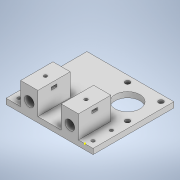
# Autodesk Inventor part: HalterungMotorNeu
Saved by Autodesk Inventor 2021 (Build 250183000, 183)
## iProperties
Created: 2021-02-28
Part Number: HalterungMotorNeu
Material: Generisch
Document SubType Name: Modeling
Designer: Elena
Density: 1 g/cm^3
Appearance: Vorgabe
Author: Elena
Autodesk Inventor part; units mm, degrees
ref_plane "YZ Plane" through (0, 0, 0) normal (1, 0, 0) x (0, 1, 0)
ref_plane "XZ Plane" through (0, 0, 0) normal (0, 1, 0) x (-1, 0, 0)
ref_plane "XY Plane" through (0, 0, 0) normal (0, 0, 1) x (1, 0, 0)
sketch "Skizze1" plane through (0, 0, 0) normal (0, 1, 0) x (-1, 0, 0)
  line L0 (0, 0) -> (65.65, 0)
  line L1 (65.65, 0) -> (65.65, -80)
  line L2 (65.65, -80) -> (0, -80)
  line L3 (0, -80) -> (0, 0)
  dimension "d0" = 65.65
  dimension "d1" = 80
  constraints: 8 end point, 2 parallel, 1 horizontal, 1 perpendicular
  measures "d0" distance of L1.end L2.end
  measures "d1" distance of L0.end L1.end
extrude "Extrusion1" add sketch "Skizze1" along normal blind 5
sketch "Skizze2" plane through (0, 5, 0) normal (0, 1, 0) x (1, 0, 0)
  line L0 (-65.65, 80) -> (-65.65, 0) projected
  line L1 (-65.65, 0) -> (0, 0) projected
  line L2 (-65.65, 0) -> (-59.65, 0) construction
  line L3 (-59.65, 0) -> (-59.65, 30)
  line L4 (-59.65, 30) -> (-43.65, 30)
  line L5 (-43.65, 30) -> (-43.65, 0)
  line L6 (-43.65, 0) -> (-59.65, 0)
  line L7 (-22, 0) -> (-22, 30)
  line L8 (-22, 30) -> (-6, 30)
  line L9 (-6, 30) -> (-6, 0)
  line L10 (-6, 0) -> (-22, 0)
  dimension "d4" = 6
  dimension "d6" = 30
  dimension "d7" = 16
  dimension "d8" = 90
  dimension "d9" = 16
  dimension "d10" = 21.65
  dimension "d11" = 30
  dimension "d12" = 16
  dimension "d13" = 90
  dimension "d14" = 30
  dimension "d15" = 90
  constraints: 18 end point, 5 perpendicular, 2 point on line, 1 collinear, 1 horizontal
  measures "d4" distance of L0.end L3.start
  measures "d6" distance of L3.start L3.end
  measures "d7" distance of L3.end L4.end
  measures "d8" angle of L3 L4
  measures "d9" distance of L5.end L3.start
  measures "d10" distance of L5.end L7.start
  measures "d11" distance of L7.start L7.end
  measures "d12" distance of L7.end L8.end
  measures "d13" angle of L7 L8
  measures "d14" distance of L8.end L9.end
  measures "d15" angle of L8 L9
extrude "Extrusion2" add sketch "Skizze2" along normal blind 21 contours L3 L4 L5 L1
sketch "Skizze3" plane through (0, 5, 0) normal (0, 1, 0) x (1, 0, 0)
  line L0 (-43.65, 0) -> (0, 0) projected
  line L1 (-43.65, 0) -> (-22, 0)
  line L2 (-22, 0) -> (-22, 30)
  line L3 (-22, 30) -> (-6, 30)
  line L4 (-6, 30) -> (-6, 0)
  line L5 (-6, 0) -> (-22, 0)
  dimension "d18" = 21.65
  dimension "d19" = 30
  dimension "d21" = 16
  dimension "d22" = 16
  constraints: 10 end point, 2 perpendicular, 2 point on line, 1 collinear, 1 horizontal
  measures "d18" distance of L0.start L1.end
  measures "d19" distance of L1.end L2.end
  measures "d21" distance of L2.end L3.end
  measures "d22" distance of L4.end L1.end
extrude "Extrusion3" add sketch "Skizze3" along normal blind 21
sketch "Skizze4" plane through (0, 5, 0) normal (0, 1, 0) x (1, 0, 0)
  line L0 (-65.65, 0) -> (0, 0) projected
  line L1 (-5.9719, 0) -> (14.5281, 0)
  line L2 (14.5281, 0) -> (14.5281, 80)
  line L3 (0, 0) -> (0, 80) projected
  line L4 (14.5281, 80) -> (0, 80)
  line L5 (0, 80) -> (0, 0)
  dimension "d25" = 20.5
  dimension "d26" = 80
  dimension "d27" = 90
  constraints: 8 end point, 2 perpendicular, 1 collinear, 1 point on line
  measures "d25" distance of L1.start L1.end
  measures "d26" distance of L1.end L2.end
  measures "d27" angle of L2 L1
extrude "Extrusion4" add sketch "Skizze4" against normal blind 5
sketch "Skizze5" plane through (0, 5, 0) normal (0, 1, 0) x (1, 0, 0)
  line L0 (-22, 30) -> (-6, 30) projected
  line L1 (-22, 30) -> (-14, 30)
  line L2 (-14, 30) -> (-14, 38)
  line L3 (-14, 38) -> (-29.5, 38)
  circle A0 centre (-29.5, 38) radius 1
  point P0 (0, 0)
  dimension "d30" = 8
  dimension "d31" = 8
  dimension "d32" = 15.5
  dimension "d33" = 2
  constraints: 6 end point, 2 perpendicular, 1 centre point, 1 coincident, 1 midpoint
  measures "d30" distance of L0.start L1.end
  measures "d31" distance of L1.end L2.end
  measures "d32" distance of L2.end L3.end
  measures "d33" diameter of A0
extrude "Extrusion5" cut sketch "Skizze5" against normal blind 5
sketch "Skizze6" plane through (0, 5, 0) normal (0, 1, 0) x (1, 0, 0)
  circle A0 centre (-29.5, 38) radius 1 projected
  line L0 (-29.5, 38) -> (1.5, 38)
  line L1 (-29.5, 38) -> (1.5, 38) construction
  circle A1 centre (1.5, 38) radius 1
  point P0 (0, 0)
  dimension "d36" = 31
  dimension "d37" = 0
  dimension "d38" = 2
  constraints: 4 end point, 2 horizontal, 1 centre point, 1 coincident, 1 collinear
  measures "d36" distance of L0.start L0.end
  measures "d37" distance between parallel lines of L0 L1
  measures "d38" diameter of A1
extrude "Extrusion6" cut sketch "Skizze6" against normal blind 5 contours A1
sketch "Skizze7" plane through (0, 5, 0) normal (0, 1, 0) x (1, 0, 0)
  circle A0 centre (1.5, 38) radius 1 projected
  line L0 (1.5, 38) -> (1.5, 69)
  circle A1 centre (1.5, 69) radius 1
  point P0 (0, 0)
  dimension "d41" = 31
  dimension "d42" = 2
  constraints: 2 end point, 1 centre point, 1 coincident, 1 vertical
  measures "d41" distance of L0.start L0.end
  measures "d42" diameter of A1
extrude "Extrusion7" cut sketch "Skizze7" against normal blind 5 contours A1
sketch "Skizze8" plane through (0, 5, 0) normal (0, 1, 0) x (1, 0, 0)
  circle A0 centre (-29.5, 38) radius 1 projected
  line L0 (-29.5, 38) -> (-29.5, 69)
  circle A1 centre (-29.5, 69) radius 1
  point P0 (0, 0)
  dimension "d45" = 31
  dimension "d46" = 2
  constraints: 2 end point, 1 centre point, 1 coincident, 1 vertical
  measures "d45" distance of L0.start L0.end
  measures "d46" diameter of A1
extrude "Extrusion8" cut sketch "Skizze8" against normal blind 5 contours A1
sketch "Skizze9" plane through (0, 5, 0) normal (0, 1, 0) x (1, 0, 0)
  circle A0 centre (1.5, 38) radius 1 projected
  line L0 (1.5, 38) -> (7.5, 38)
  line L1 (14.5281, 80) -> (-65.65, 80) projected
  line L2 (-65.65, 0) -> (14.5281, 0) projected
  line L3 (14.5281, 0) -> (14.5281, 80) projected
  line L4 (7.5, 38) -> (14.5281, 38)
  line L5 (14.5281, 38) -> (14.5281, 80)
  line L6 (14.5281, 80) -> (7.5, 80)
  line L7 (7.5, 80) -> (7.5, 38)
  point P0 (0, 0)
  dimension "d49" = 6
  constraints: 10 end point, 2 horizontal, 2 parallel, 1 perpendicular
  measures "d49" distance of L0.start L0.end
extrude "Extrusion9" cut sketch "Skizze9" against normal blind 5 contours L7 L1 L3 L4
sketch "Skizze10" plane through (0, 5, 0) normal (0, 1, 0) x (1, 0, 0)
  line L0 (7.5, 38) -> (7.5, 80) projected
  line L1 (14.5281, 0) -> (14.5281, 38) projected
  line L2 (7.5, 38) -> (14.5281, 38)
  line L3 (14.5281, 38) -> (14.5281, 0)
  line L4 (14.5281, 0) -> (7.5, 0)
  line L5 (7.5, 0) -> (7.5, 38)
  point P0 (0, 0)
  constraints: 8 end point, 2 parallel, 1 horizontal, 1 perpendicular
extrude "Extrusion10" cut sketch "Skizze10" against normal blind 5
sketch "Skizze11" plane through (0, 5, 0) normal (0, 1, 0) x (1, 0, 0)
  circle A0 centre (1.5, 69) radius 1 projected
  line L0 (1.5, 69) -> (1.5, 75)
  line L1 (1.5, 75) -> (7.5, 75)
  line L2 (7.5, 0) -> (7.5, 80) projected
  line L3 (7.5, 80) -> (1.5, 80)
  line L4 (7.5, 80) -> (-65.65, 80) projected
  line L5 (1.5, 75) -> (1.5, 80)
  point P0 (0, 0)
  dimension "d54" = 6
  constraints: 8 end point, 3 point on line, 2 perpendicular, 1 vertical
  measures "d54" distance of L0.start L0.end
extrude "Extrusion11" cut sketch "Skizze11" against normal blind 5 contours L5 L3 L2 L1
sketch "Skizze12" plane through (0, 5, 0) normal (0, 1, 0) x (1, 0, 0)
  line L0 (1.5, 80) -> (-65.65, 80) projected
  line L1 (1.5, 75) -> (-65.65, 75)
  line L2 (-65.65, 75) -> (-65.65, 80)
  line L3 (-65.65, 80) -> (1.5, 80)
  line L4 (1.5, 80) -> (1.5, 75)
  point P0 (0, 0)
  constraints: 8 end point, 2 parallel, 1 horizontal, 1 perpendicular
extrude "Extrusion12" cut sketch "Skizze12" against normal blind 5
sketch "Skizze13" plane through (0, 5, 0) normal (0, 1, 0) x (1, 0, 0)
  circle A0 centre (1.5, 38) radius 1 projected
  line L0 (1.5, 38) -> (1.5, 23)
  circle A1 centre (1.5, 23) radius 1
  point P0 (0, 0)
  dimension "d59" = 15
  dimension "d60" = 2
  constraints: 2 end point, 1 centre point, 1 coincident, 1 vertical
  measures "d59" distance of L0.start L0.end
  measures "d60" diameter of A1
extrude "Extrusion13" cut sketch "Skizze13" against normal blind 5 contours A1
sketch "Skizze14" plane through (0, 5, 0) normal (0, 1, 0) x (1, 0, 0)
  circle A0 centre (1.5, 23) radius 1 projected
  line L0 (-65.65, 0) -> (7.5, 0) projected
  line L1 (-6, 30) -> (-6, 0) projected
  line L2 (1.5, 0) -> (-6, 0)
  line L3 (1.5, 0) -> (1.5, 6)
  circle A1 centre (1.5, 6) radius 1
  point P0 (0, 0)
  dimension "d63" = 6
  dimension "d64" = 2
  constraints: 4 end point, 1 centre point, 1 coincident, 1 horizontal, 1 point on line, 1 vertical
  measures "d63" distance of L2.start L3.end
  measures "d64" diameter of A1
extrude "Extrusion14" cut sketch "Skizze14" against normal blind 5 contours A1
sketch "Skizze15" plane through (0, 5, 0) normal (0, 1, 0) x (1, 0, 0)
  line L0 (-65.65, 0) -> (7.5, 0) projected
  line L1 (-65.65, 0) -> (-62.65, 0)
  line L2 (-62.65, 0) -> (-62.65, 6)
  circle A0 centre (-62.65, 6) radius 1
  point P0 (0, 0)
  dimension "d67" = 3
  dimension "d68" = 6
  dimension "d69" = 2
  constraints: 4 end point, 1 centre point, 1 coincident, 1 perpendicular, 1 point on line
  measures "d67" distance of L0.start L1.end
  measures "d68" distance of L1.end L2.end
  measures "d69" diameter of A0
extrude "Extrusion15" cut sketch "Skizze15" against normal blind 5
sketch "Skizze16" plane through (0, 5, 0) normal (0, 1, 0) x (1, 0, 0)
  circle A0 centre (-62.65, 6) radius 1 projected
  line L0 (-62.65, 6) -> (-62.65, 23)
  circle A1 centre (-62.65, 23) radius 1
  point P0 (0, 0)
  dimension "d72" = 17
  dimension "d73" = 2
  constraints: 2 end point, 1 centre point, 1 coincident, 1 vertical
  measures "d72" distance of L0.start L0.end
  measures "d73" diameter of A1
extrude "Extrusion16" cut sketch "Skizze16" against normal blind 5 contours A1
sketch "Skizze17" plane through (-65.65, 0, 0) normal (0, 0, 1) x (1, 0, 0)
  line L0 (6, 26) -> (22, 26) projected
  line L1 (6, 26) -> (14, 26)
  line L2 (14, 26) -> (14, 13)
  circle A0 centre (14, 13) radius 4.5
  point P0 (65.65, 0)
  dimension "d76" = 8
  dimension "d77" = 13
  dimension "d78" = 9
  constraints: 4 end point, 1 centre point, 1 coincident, 1 midpoint, 1 perpendicular
  measures "d76" distance of L0.start L1.end
  measures "d77" distance of L1.end L2.end
  measures "d78" diameter of A0
extrude "Extrusion17" cut sketch "Skizze17" against normal blind 30
sketch "Skizze18" plane through (-65.65, 0, 0) normal (0, 0, 1) x (1, 0, 0)
  line L0 (43.65, 5) -> (43.65, 26) projected
  line L1 (43.65, 26) -> (51.65, 26)
  line L2 (51.65, 26) -> (51.65, 13)
  circle A0 centre (51.65, 13) radius 4.5
  point P0 (65.65, 0)
  dimension "d81" = 8
  dimension "d82" = 13
  dimension "d83" = 9
  constraints: 4 end point, 1 centre point, 1 coincident, 1 horizontal, 1 perpendicular
  measures "d81" distance of L0.end L1.end
  measures "d82" distance of L1.end L2.end
  measures "d83" diameter of A0
extrude "Extrusion18" cut sketch "Skizze18" against normal blind 30
sketch "Skizze19" plane through (-59.65, 5, -30) normal (-1, 0, 0) x (0, 0, 1)
  line L0 (0, 0) -> (0, 21) projected
  line L1 (0, 21) -> (15, 21)
  line L2 (0, 21) -> (30, 21) projected
  line L3 (15, 21) -> (15, 17)
  line L4 (15, 17) -> (17.75, 17)
  line L5 (17.75, 17) -> (12.25, 17)
  line L6 (12.25, 17) -> (12.25, 15.75)
  line L7 (12.25, 15.75) -> (17.75, 15.75)
  line L8 (17.75, 15.75) -> (17.75, 17)
  point P0 (30, -5)
  dimension "d86" = 15
  dimension "d87" = 4
  dimension "d88" = 2.75
  dimension "d89" = 5.5
  dimension "d90" = 1.25
  constraints: 14 end point, 3 perpendicular, 2 parallel, 1 horizontal, 1 midpoint
  measures "d86" distance of L0.end L1.end
  measures "d87" distance of L1.end L3.end
  measures "d88" distance of L3.end L4.end
  measures "d89" distance of L7.end L6.end
  measures "d90" distance of L6.end L5.end
extrude "Extrusion19" cut sketch "Skizze19" against normal blind 16
sketch "Skizze20" plane through (0, 5, 0) normal (0, 1, 0) x (1, 0, 0)
  circle A0 centre (1.5, 23) radius 1 projected
  circle A1 centre (1.5, 23) radius 1.5
  point P0 (0, 0)
  dimension "d93" = 3
  constraints: 1 centre point, 1 coincident
  measures "d93" diameter of A1
extrude "Extrusion20" cut sketch "Skizze20" against normal blind 5 contours A0 | A1
sketch "Skizze21" plane through (0, 5, 0) normal (0, 1, 0) x (1, 0, 0)
  circle A0 centre (1.5, 6) radius 1 projected
  circle A1 centre (1.5, 6) radius 1.5
  point P0 (0, 0)
  dimension "d96" = 3
  constraints: 1 centre point, 1 coincident
  measures "d96" diameter of A1
extrude "Extrusion21" cut sketch "Skizze21" against normal blind 5 contours A0 | A1
sketch "Skizze22" plane through (0, 5, 0) normal (0, 1, 0) x (1, 0, 0)
  circle A0 centre (-62.65, 23) radius 1 projected
  circle A1 centre (-62.65, 23) radius 1.5
  point P0 (0, 0)
  dimension "d99" = 3
  constraints: 1 centre point, 1 coincident
  measures "d99" diameter of A1
extrude "Extrusion22" cut sketch "Skizze22" against normal blind 5 contours A0 | A1
sketch "Skizze23" plane through (0, 5, 0) normal (0, 1, 0) x (1, 0, 0)
  circle A0 centre (-62.65, 6) radius 1 projected
  circle A1 centre (-62.65, 6) radius 1.5
  point P0 (0, 0)
  dimension "d102" = 3
  constraints: 1 centre point, 1 coincident
  measures "d102" diameter of A1
extrude "Extrusion23" cut sketch "Skizze23" against normal blind 5 contours A0 | A1
sketch "Skizze24" plane through (0, 5, 0) normal (0, 1, 0) x (1, 0, 0)
  circle A0 centre (1.5, 69) radius 1 projected
  circle A1 centre (1.5, 69) radius 2.25
  point P0 (0, 0)
  dimension "d105" = 4.5
  constraints: 1 centre point, 1 coincident
  measures "d105" diameter of A1
extrude "Extrusion24" cut sketch "Skizze24" against normal blind 5 contours A0 | A1
sketch "Skizze25" plane through (0, 5, 0) normal (0, 1, 0) x (1, 0, 0)
  circle A0 centre (-29.5, 69) radius 1 projected
  circle A1 centre (-29.5, 69) radius 2.25
  point P0 (0, 0)
  dimension "d108" = 4.5
  constraints: 1 centre point, 1 coincident
  measures "d108" diameter of A1
extrude "Extrusion25" cut sketch "Skizze25" against normal blind 5 contours A0 | A1
sketch "Skizze26" plane through (0, 5, 0) normal (0, 1, 0) x (1, 0, 0)
  circle A0 centre (1.5, 38) radius 1 projected
  circle A1 centre (1.5, 38) radius 2.25
  point P0 (0, 0)
  dimension "d112" = 4.5
  constraints: 1 centre point, 1 coincident
  measures "d112" diameter of A1
extrude "Extrusion26" cut sketch "Skizze26" against normal blind 5 contours A0 | A1
sketch "Skizze27" plane through (0, 5, 0) normal (0, 1, 0) x (1, 0, 0)
  circle A0 centre (-29.5, 38) radius 1 projected
  circle A1 centre (-29.5, 38) radius 2.25
  point P0 (0, 0)
  dimension "d115" = 4.5
  constraints: 1 centre point, 1 coincident
  measures "d115" diameter of A1
extrude "Extrusion27" cut sketch "Skizze27" against normal blind 5 contours A0 | A1
sketch "Skizze28" plane through (0, 26, 0) normal (0, 1, 0) x (1, 0, 0)
  line L0 (-43.65, 30) -> (-43.65, 0) projected
  line L1 (-59.65, 0) -> (-59.65, 30) projected
  line L2 (-43.65, 0) -> (-59.65, 30)
  line L3 (-59.65, 30) -> (-43.65, 30) projected
  line L4 (-43.65, 30) -> (-59.65, 0)
  circle A0 centre (-51.65, 15) radius 1.5
  point P0 (0, 0)
  dimension "d118" = 3
  constraints: 4 end point, 1 centre point, 1 midpoint
  measures "d118" diameter of A0
extrude "Extrusion28" cut sketch "Skizze28" against normal blind 13 contours A0 L2 L4 | L4 L2 A0 | A0 L4 L2 | L2 L4 A0
sketch "Skizze29" plane through (-6, 5, 0) normal (1, 0, 0) x (0, 0, -1)
  line L0 (0, 21) -> (15, 21)
  line L1 (0, 21) -> (30, 21) projected
  line L2 (15, 21) -> (11, 21)
  line L3 (15, 21) -> (15, 17)
  line L4 (15, 21) -> (19, 21) construction
  line L5 (15, 17) -> (17.27, 17)
  line L6 (12.25, 17) -> (17.75, 17) projected
  line L7 (17.27, 17) -> (11.77, 17)
  line L8 (11.77, 17) -> (11.77, 15.75)
  line L9 (11.77, 15.75) -> (17.27, 15.75)
  line L10 (17.27, 15.75) -> (17.27, 17)
  point P0 (0, -5)
  dimension "d123" = 15
  dimension "d124" = 4
  dimension "d125" = 4
  dimension "d126" = 90
  dimension "d127" = 2.27
  dimension "d128" = 5.5
  dimension "d129" = 1.25
  constraints: 18 end point, 2 horizontal, 2 parallel, 2 perpendicular, 2 point on line, 1 midpoint, 1 vertical
  measures "d123" distance of L0.start L0.end
  measures "d124" distance of L0.end L2.end
  measures "d125" distance of L0.end L3.end
  measures "d126" angle of L3 L4
  measures "d127" distance of L3.end L5.end
  measures "d128" distance of L9.end L8.end
  measures "d129" distance of L8.end L7.end
extrude "Extrusion29" cut sketch "Skizze29" against normal blind 16
sketch "Skizze30" plane through (0, 26, 0) normal (0, 1, 0) x (1, 0, 0)
  line L0 (-22, 30) -> (-22, 0) projected
  line L1 (-6, 0) -> (-6, 30) projected
  line L2 (-22, 0) -> (-6, 30)
  line L3 (-22, 30) -> (-6, 0)
  circle A0 centre (-14, 15) radius 1.5
  point P0 (0, 0)
  dimension "d132" = 3
  constraints: 4 end point, 1 centre point, 1 midpoint
  measures "d132" diameter of A0
extrude "Extrusion30" cut sketch "Skizze30" against normal blind 13 contours A0 L2 L3 | L3 L2 A0 | L2 L3 A0 | L2 A0 L3
sketch "Skizze31" plane through (0, 5, 0) normal (0, 1, 0) x (1, 0, 0)
  circle A0 centre (-29.5, 38) radius 2.25 projected
  circle A1 centre (1.5, 69) radius 2.25 projected
  line L0 (-29.5, 38) -> (1.5, 69)
  circle A2 centre (-29.5, 69) radius 2.25 projected
  circle A3 centre (1.5, 38) radius 2.25 projected
  line L1 (-29.5, 69) -> (1.5, 38)
  circle A4 centre (-14, 53.5) radius 11.5
  point P0 (0, 0)
  dimension "d137" = 23
  constraints: 4 end point, 1 centre point, 1 midpoint
  measures "d137" diameter of A4
extrude "Extrusion31" cut sketch "Skizze31" against normal blind 5 contours A4 L1 L0 | L0 L1 A4 | L1 A4 L0 | L0 A4 L1
sketch "Skizze32" plane through (0, 5, 0) normal (0, 1, 0) x (1, 0, 0)
  point P0 (0, 0)
sketch "Skizze33" plane through (0, 5, 0) normal (0, 1, 0) x (1, 0, 0)
  circle A0 centre (-62.65, 6) radius 1.5 projected
  circle A1 centre (-62.65, 6) radius 1.5
  point P0 (0, 0)
  dimension "d140" = 3
  constraints: 1 centre point, 1 coincident
  measures "d140" diameter of A1
extrude "Extrusion32" add sketch "Skizze33" against normal blind 5
sketch "Skizze34" plane through (0, 5, 0) normal (0, 1, 0) x (1, 0, 0)
  circle A0 centre (-62.65, 23) radius 1.5 projected
  circle A1 centre (-62.65, 23) radius 1.5
  point P0 (0, 0)
  dimension "d143" = 3
  constraints: 1 centre point, 1 coincident
  measures "d143" diameter of A1
extrude "Extrusion33" add sketch "Skizze34" against normal blind 5
sketch "Skizze35" plane through (0, 5, 0) normal (0, 1, 0) x (1, 0, 0)
  line L0 (-59.65, 0) -> (-59.65, 30) projected
  line L1 (-59.65, 0) -> (-73.15, 0)
  line L2 (-65.65, 0) -> (-59.65, 0) projected
  line L3 (-65.65, 0) -> (7.5, 0) projected
  line L4 (-65.65, 0) -> (-73.15, 0)
  line L5 (-73.15, 0) -> (-73.15, 75)
  line L6 (-73.15, 75) -> (-65.65, 75)
  line L7 (-65.65, 75) -> (-65.65, 0)
  point P0 (0, 0)
  dimension "d146" = 13.5
  dimension "d147" = 75
  constraints: 10 end point, 2 parallel, 1 collinear, 1 horizontal, 1 perpendicular
  measures "d146" distance of L0.start L1.end
  measures "d147" distance of L4.end L5.end
extrude "Extrusion34" add sketch "Skizze35" against normal blind 5
sketch "Skizze36" plane through (0, 5, 0) normal (0, 1, 0) x (1, 0, 0)
  line L0 (-73.15, 0) -> (-73.15, 75) projected
  line L1 (-73.15, 0) -> (-67.15, 0)
  line L2 (-67.15, 0) -> (-67.15, 6)
  line L3 (-67.15, 6) -> (-73.15, 6)
  line L4 (-73.15, 6) -> (-73.15, 0)
  circle A0 centre (-67.15, 6) radius 1.5
  point P0 (0, 0)
  dimension "d150" = 6
  dimension "d151" = 6
  dimension "d152" = 3
  constraints: 8 end point, 2 parallel, 1 centre point, 1 coincident, 1 horizontal, 1 perpendicular
  measures "d150" distance of L3.end L2.end
  measures "d151" distance of L2.end L1.end
  measures "d152" diameter of A0
extrude "Extrusion35" cut sketch "Skizze36" against normal blind 5 contours A0 L2 L3 | L3 L2 A0
sketch "Skizze37" plane through (0, 5, 0) normal (0, 1, 0) x (1, 0, 0)
  circle A0 centre (-67.15, 6) radius 1.5 projected
  line L0 (-67.15, 6) -> (-67.15, 23)
  circle A1 centre (-67.15, 23) radius 1.5
  point P0 (0, 0)
  dimension "d155" = 17
  dimension "d156" = 3
  constraints: 2 end point, 1 centre point, 1 coincident, 1 vertical
  measures "d155" distance of L0.start L0.end
  measures "d156" diameter of A1
extrude "Extrusion36" cut sketch "Skizze37" against normal blind 5 contours A1
sketch "Skizze38" plane through (-6, 5, 0) normal (1, 0, 0) x (0, 0, -1)
  line L0 (17.27, 17) -> (11.77, 17) projected
  line L1 (11.77, 17) -> (11.77, 17.625)
  line L2 (11.77, 17.625) -> (17.27, 17.625)
  line L3 (17.27, 17.625) -> (17.27, 17)
  line L4 (12.25, 17) -> (17.75, 17) projected
  point P0 (0, -5)
  dimension "d159" = 0.625
  dimension "d160" = 5.5
  dimension "d161" = 90
  constraints: 6 end point, 2 perpendicular, 1 point on line, 1 vertical
  measures "d159" distance of L0.end L1.end
  measures "d160" distance of L1.end L2.end
  measures "d161" angle of L1 L2
extrude "Extrusion37" cut sketch "Skizze38" against normal blind 16
sketch "Skizze39" plane through (-6, 5, 0) normal (1, 0, 0) x (0, 0, -1)
  line L0 (17.27, 15.75) -> (11.77, 15.75) projected
  line L1 (11.77, 15.75) -> (17.27, 15.75)
  line L2 (17.27, 15.75) -> (17.27, 15.125)
  line L3 (17.27, 15.125) -> (11.77, 15.125)
  line L4 (11.77, 15.125) -> (11.77, 15.75)
  point P0 (0, -5)
  dimension "d164" = 5.5
  dimension "d165" = 0.625
  constraints: 8 end point, 2 parallel, 1 horizontal, 1 perpendicular
  measures "d164" distance of L2.end L3.end
  measures "d165" distance of L1.end L2.end
extrude "Extrusion38" cut sketch "Skizze39" against normal blind 16
sketch "Skizze40" plane through (-59.65, 5, -30) normal (-1, 0, 0) x (0, 0, 1)
  line L0 (12.73, 17.625) -> (18.23, 17.625) projected
  line L1 (12.25, 17) -> (17.75, 17)
  line L2 (17.75, 17) -> (17.75, 17.625)
  line L3 (17.75, 17.625) -> (12.25, 17.625)
  line L4 (12.25, 17.625) -> (12.25, 17)
  point P0 (30, -5)
  dimension "d168" = 5.5
  constraints: 8 end point, 2 parallel, 1 horizontal, 1 perpendicular, 1 point on line
  measures "d168" distance of L3.end L2.end
extrude "Extrusion39" cut sketch "Skizze40" against normal blind 16
sketch "Skizze41" plane through (-59.65, 5, -30) normal (-1, 0, 0) x (0, 0, 1)
  line L0 (12.25, 15.75) -> (17.75, 15.75) projected
  line L1 (12.25, 15.75) -> (17.75, 15.75)
  line L2 (17.75, 15.75) -> (17.75, 15.125)
  line L3 (17.75, 15.125) -> (12.25, 15.125)
  line L4 (12.25, 15.125) -> (12.25, 15.75)
  point P0 (30, -5)
  dimension "d171" = 5.5
  dimension "d172" = 0.625
  constraints: 8 end point, 2 parallel, 1 horizontal, 1 perpendicular
  measures "d171" distance of L2.end L3.end
  measures "d172" distance of L1.end L2.end
extrude "Extrusion40" cut sketch "Skizze41" against normal blind 16
sketch "Skizze42" plane through (-6, 5, 0) normal (1, 0, 0) x (0, 0, -1)
  line L0 (11.77, 17.625) -> (11.77, 15.125) projected
  line L1 (17.75, 15.125) -> (12.25, 15.125) projected
  line L2 (11.77, 17.625) -> (17.27, 17.625)
  line L3 (17.27, 17.625) -> (17.27, 15.125)
  line L4 (17.27, 15.125) -> (11.77, 15.125)
  line L5 (11.77, 15.125) -> (11.77, 17.625)
  point P0 (0, -5)
  dimension "d175" = 5.5
  constraints: 8 end point, 2 parallel, 1 horizontal, 1 perpendicular, 1 point on line
  measures "d175" distance of L3.end L4.end
extrude "Extrusion41" add sketch "Skizze42" against normal blind 16
sketch "Skizze43" plane through (0, 26, 0) normal (0, 1, 0) x (1, 0, 0)
  circle A0 centre (-14, 15) radius 1.5 projected
  line L0 (-14, 15) -> (-6, 15)
  line L1 (-6, 0) -> (-6, 30) projected
  point P0 (0, 0)
  constraints: 2 end point, 1 midpoint
sketch "Skizze44" plane through (-6, 5, 0) normal (1, 0, 0) x (0, 0, -1)
  line L0 (0, 21) -> (30, 21) projected
  line L1 (15, 21) -> (15, 17.5)
  line L2 (15, 17.5) -> (17.55, 17.5)
  line L3 (17.55, 17.5) -> (17.55, 15)
  line L4 (17.55, 15) -> (12.45, 15)
  line L5 (12.45, 15) -> (12.45, 17.5)
  line L6 (12.45, 17.5) -> (15, 17.5)
  point P0 (0, -5)
  dimension "d178" = 3.5
  dimension "d179" = 2.55
  dimension "d180" = 2.5
  dimension "d181" = 90
  dimension "d182" = 5.1
  dimension "d183" = 2.5
  constraints: 12 end point, 3 perpendicular, 1 midpoint, 1 point on line, 1 vertical
  measures "d178" distance of L1.start L1.end
  measures "d179" distance of L1.end L2.end
  measures "d180" distance of L2.end L3.end
  measures "d181" angle of L2 L3
  measures "d182" distance of L3.end L4.end
  measures "d183" distance of L4.end L5.end
extrude "Extrusion42" cut sketch "Skizze44" against normal blind 16
sketch "Skizze45" plane through (0, 26, 0) normal (0, 1, 0) x (1, 0, 0)
  circle A0 centre (-14, 15) radius 1.5 projected
  circle A1 centre (-14, 15) radius 1.5
  point P0 (0, 0)
  dimension "d186" = 3
  constraints: 1 centre point, 1 coincident
  measures "d186" diameter of A1
extrude "Extrusion43" add sketch "Skizze45" against normal blind 3.6
extrude "Extrusion44" cut sketch "Skizze43" against normal blind 3.6
sketch "Skizze46" plane through (-59.65, 5, -30) normal (-1, 0, 0) x (0, 0, 1)
  line L0 (12.25, 17.625) -> (12.25, 15.125) projected
  line L1 (12.25, 15.125) -> (17.75, 15.125) projected
  line L2 (12.25, 17.625) -> (17.75, 17.625)
  line L3 (17.75, 17.625) -> (17.75, 15.125)
  line L4 (17.75, 15.125) -> (12.25, 15.125)
  line L5 (12.25, 15.125) -> (12.25, 17.625)
  point P0 (30, -5)
  constraints: 8 end point, 2 parallel, 1 horizontal, 1 perpendicular
extrude "Extrusion45" add sketch "Skizze46" against normal blind 16
sketch "Skizze47" plane through (0, 26, 0) normal (0, 1, 0) x (1, 0, 0)
  circle A0 centre (-51.65, 15) radius 1.5 projected
  line L0 (-51.65, 15) -> (-59.65, 15)
  line L1 (-59.65, 30) -> (-59.65, 0) projected
  point P0 (0, 0)
  constraints: 2 end point, 1 midpoint
sketch "Skizze48" plane through (-59.65, 5, -30) normal (-1, 0, 0) x (0, 0, 1)
  line L0 (0, 21) -> (30, 21) projected
  line L1 (15, 21) -> (15, 17.5)
  line L2 (15, 21) -> (18.5, 21) construction
  line L3 (15, 17.5) -> (17.55, 17.5)
  line L4 (17.55, 17.5) -> (17.55, 15)
  line L5 (17.55, 15) -> (12.45, 15)
  line L6 (12.45, 15) -> (12.45, 17.5)
  line L7 (12.45, 17.5) -> (15, 17.5)
  point P0 (30, -5)
  dimension "d193" = 3.5
  dimension "d194" = 90
  dimension "d195" = 2.55
  dimension "d196" = 2.5
  dimension "d197" = 5.1
  dimension "d198" = 2.5
  constraints: 14 end point, 4 perpendicular, 1 horizontal, 1 midpoint, 1 point on line, 1 vertical
  measures "d193" distance of L1.start L1.end
  measures "d194" angle of L1 L2
  measures "d195" distance of L1.end L3.end
  measures "d196" distance of L3.end L4.end
  measures "d197" distance of L4.end L5.end
  measures "d198" distance of L5.end L6.end
extrude "Extrusion46" cut sketch "Skizze48" against normal blind 16
sketch "Skizze49" plane through (0, 26, 0) normal (0, 1, 0) x (1, 0, 0)
  circle A0 centre (-51.65, 15) radius 1.5 projected
  circle A1 centre (-51.65, 15) radius 1.5
  point P0 (0, 0)
  dimension "d201" = 3
  constraints: 1 centre point, 1 coincident
  measures "d201" diameter of A1
extrude "Extrusion47" add sketch "Skizze49" against normal blind 3.6
extrude "Extrusion48" cut sketch "Skizze47" against normal blind 3.6
